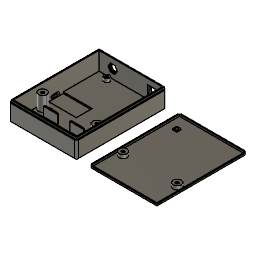
enclosure_tx (Autodesk Fusion 360 design; units mm, degrees)
part number: 2026-03-28-19-02-26-075
Autodesk Fusion 360 part; units mm, degrees
sketch "Sketch6" plane through (0, 0, 0) normal (0, 0, 1) x (1, 0, 0)
  line L0 (0, -4) -> (65, -4)
  line L1 (65, -4) -> (65, -22.2)
  line L2 (65, -22.2) -> (0, -22.2)
  line L3 (0, -22.2) -> (0, -4)
  line L4 (7.5, 70) -> (57.5, 70)
  line L5 (57.5, 70) -> (57.5, 0)
  line L6 (57.5, 0) -> (7.5, 0)
  line L7 (7.5, 0) -> (7.5, 70)
  line L8 (-5, 73) -> (70, 73)
  line L9 (70, 73) -> (70, -27)
  line L10 (70, -27) -> (-5, -27)
  line L11 (-5, -27) -> (-5, 73)
  dimension "d33" = 18.2
  dimension "d35" = 65
  dimension "d36" = 50
  dimension "d37" = 70
  dimension "d38" = 4
  dimension "d39" = 7.5
  dimension "d40" = 75
  dimension "d41" = 100
  dimension "d42" = 3
  dimension "d43" = 12.5
  constraint horizontal L0
  constraint vertical L1
  constraint horizontal L2
  constraint vertical L3
  constraint horizontal L4
  constraint vertical L5
  constraint horizontal L6
  constraint vertical L7
  constraint horizontal L8
  constraint vertical L9
  constraint horizontal L10
  constraint vertical L11
  measures "d33" distance of L0.start L2.end
  measures "d35" distance of L1.end L2.end
  measures "d36" distance of L4.start L4.end
  measures "d37" distance of L4.start L6.end
  measures "d38" distance of L0 L6
  measures "d39" distance of L3 L7
  measures "d40" distance of L8.start L8.end
  measures "d41" distance of L8.start L10.end
  measures "d42" distance of L4 L8
  measures "d43" distance of L7 L11
extrude "Extrude9" add sketch "Sketch6" along normal blind 22 contours L0 L1 L2 L3 | L4 L5 L6 L7 | L8 L9 L10 L11 makes body 1
sketch "Sketch7" plane through (0, 0, 22) normal (0, 0, 1) x (-1, 0, 0)
  line L0 (5, 27) -> (-70, 27)
  line L1 (-70, 27) -> (-70, -73)
  line L2 (-70, -73) -> (5, -73)
  line L3 (5, -73) -> (5, 27)
  line L4 (2.5, -70.5) -> (-67.5, -70.5)
  line L5 (-67.5, -70.5) -> (-67.5, 24.5)
  line L6 (-67.5, 24.5) -> (2.5, 24.5)
  line L7 (2.5, 24.5) -> (2.5, -70.5)
  line L8 (5, -73) -> (-70, -73)
  line L9 (5, 27) -> (5, -73)
  dimension "d46" = 70
  dimension "d47" = 95
  dimension "d48" = 2.5
  dimension "d49" = 2.5
  constraint horizontal L4
  constraint vertical L5
  constraint horizontal L6
  constraint vertical L7
  measures "d46" distance of L4.start L4.end
  measures "d47" distance of L4.start L6.end
  measures "d48" distance of L4 L8
  measures "d49" distance of L7 L9
extrude "Extrude10" cut sketch "Sketch7" against normal blind 20 contours L4 L5 L6 L7 bodies 1
sketch "Sketch8" plane through (0, 0, 2) normal (0, 0, 1) x (-1, 0, 0)
  line L0 (2.5, 24.5) -> (-67.5, 24.5)
  line L1 (-67.5, 24.5) -> (-67.5, -70.5)
  line L2 (-67.5, -70.5) -> (2.5, -70.5)
  line L3 (2.5, -70.5) -> (2.5, 24.5)
  line L4 (-7.5, -68.5) -> (-57.5, -68.5)
  line L5 (-57.5, -68.5) -> (-57.5, 1.5)
  line L6 (-57.5, 1.5) -> (-7.5, 1.5)
  line L7 (-7.5, 1.5) -> (-7.5, -68.5)
  line L8 (2.5, 24.5) -> (2.5, -70.5)
  line L9 (0, 4.3) -> (-65, 4.3)
  line L10 (-65, 4.3) -> (-65, 22.5)
  line L11 (-65, 22.5) -> (0, 22.5)
  line L12 (0, 22.5) -> (0, 4.3)
  line L13 (2.5, -70.5) -> (-67.5, -70.5)
  line L14 (-10.5, 3.85) -> (-25.5, 3.85)
  line L15 (-25.5, 3.85) -> (-25.5, 2.35)
  line L16 (-25.5, 2.35) -> (-10.5, 2.35)
  line L17 (-10.5, 2.35) -> (-10.5, 3.85)
  line L18 (-39.5, 2.35) -> (-54.5, 2.35)
  line L19 (-54.5, 2.35) -> (-54.5, 3.85)
  line L20 (-54.5, 3.85) -> (-39.5, 3.85)
  line L21 (-39.5, 3.85) -> (-39.5, 2.35)
  line L22 (-67.5, 24.5) -> (2.5, 24.5)
  line L23 (-25.51, 22.9) -> (-40.51, 22.9)
  line L24 (-40.51, 22.9) -> (-40.51, 24.15)
  line L25 (-40.51, 24.15) -> (-25.51, 24.15)
  line L26 (-25.51, 24.15) -> (-25.51, 22.9)
  circle A0 centre (-10.8, -65.7) radius 1.5
  circle A1 centre (-54.2, -65.7) radius 1.5
  circle A2 centre (-54.2, -1.3) radius 1.5
  circle A3 centre (-10.8, -1.3) radius 1.5
  circle A4 centre (-10.8, -65.7) radius 3
  circle A5 centre (-54.2, -65.7) radius 3
  circle A6 centre (-54.2, -1.3) radius 3
  circle A7 centre (-10.8, -1.3) radius 3
  line L27 (-65, 19.4) -> (0, 19.4)
  line L28 (0, 19.4) -> (0, 7.4)
  line L29 (0, 7.4) -> (-65, 7.4)
  line L30 (-65, 7.4) -> (-65, 19.4)
  dimension "d52" = 50
  dimension "d53" = 70
  dimension "d54" = 10
  dimension "d55" = 65
  dimension "d56" = 18.2
  dimension "d57" = 2.5
  dimension "d58" = 2
  dimension "d59" = 15
  dimension "d60" = 1.5
  dimension "d61" = 0.45
  dimension "d62" = 15
  dimension "d63" = 1.5
  dimension "d64" = 0.45
  dimension "d65" = 3
  dimension "d66" = 3
  dimension "d67" = 2
  dimension "d68" = 15
  dimension "d69" = 1.25
  dimension "d70" = 0.4
  dimension "d71" = 0.01
  dimension "d72" = 1.01
  dimension "d73" = 3
  dimension "d74" = 3
  dimension "d75" = 3
  dimension "d76" = 3
  dimension "d77" = 3.3
  dimension "d78" = 2.8
  dimension "d79" = 2.8
  dimension "d80" = 2.8
  dimension "d81" = 2.8
  dimension "d82" = 3.3
  dimension "d83" = 3.3
  dimension "d84" = 3.3
  dimension "d85" = 6
  dimension "d86" = 6
  dimension "d87" = 6
  dimension "d88" = 6
  dimension "d93" = 12
  dimension "d94" = 3.1
  constraint horizontal L4
  constraint vertical L5
  constraint horizontal L6
  constraint vertical L7
  constraint horizontal L9
  constraint vertical L10
  constraint horizontal L11
  constraint vertical L12
  constraint horizontal L14
  constraint vertical L15
  constraint horizontal L16
  constraint vertical L17
  constraint horizontal L18
  constraint vertical L19
  constraint horizontal L20
  constraint vertical L21
  constraint horizontal L23
  constraint vertical L24
  constraint horizontal L25
  constraint vertical L26
  constraint concentric A0 A4
  constraint concentric A1 A5
  constraint concentric A2 A6
  constraint concentric A3 A7
  constraint horizontal L27
  constraint vertical L28
  constraint horizontal L29
  constraint vertical L30
  constraint coincident L12 L28.end
  constraint coincident L10 L27.start
  measures "d52" distance of L4.start L4.end
  measures "d53" distance of L4.start L6.end
  measures "d54" distance of L7 L8
  measures "d55" distance of L9.start L9.end
  measures "d56" distance of L9.start L11.end
  measures "d57" distance of L8 L12
  measures "d58" distance of L4 L13
  measures "d59" distance of L14.start L14.end
  measures "d60" distance of L14.start L16.end
  measures "d61" distance of L9 L14
  measures "d62" distance of L18.start L18.end
  measures "d63" distance of L18.start L20.end
  measures "d64" distance of L9 L20
  measures "d65" distance of L5 L19
  measures "d66" distance of L7 L17
  measures "d67" distance of L11 L22
  measures "d68" distance of L23.start L23.end
  measures "d69" distance of L23.start L25.end
  measures "d70" distance of L11 L23
  measures "d71" distance of L15 L26
  measures "d72" distance of L21 L24
  measures "d73" diameter of A0
  measures "d74" diameter of A1
  measures "d75" diameter of A2
  measures "d76" diameter of A3
  measures "d77" distance of L5 A1.centre
  measures "d78" distance of L4 A1.centre
  measures "d79" distance of L4 A0.centre
  measures "d80" distance of L6 A2.centre
  measures "d81" distance of L6 A3.centre
  measures "d82" distance of L7 A0.centre
  measures "d83" distance of L7 A3.centre
  measures "d84" distance of L5 A2.centre
  measures "d85" diameter of A4
  measures "d86" diameter of A5
  measures "d87" diameter of A6
  measures "d88" diameter of A7
  measures "d93" distance of L27 L29
  measures "d94" distance of L11 L27
extrude "Extrude11" add sketch "Sketch8" along normal blind 4 contours L4 A4 | L4 A4 | L6 A7 | L6 A7 | L4 A5 | L4 A5 | L6 A6 | L6 A6 bodies 1
extrude "Extrude12" add sketch "Sketch8" along normal blind 10 contours L14 L15 L16 L17 | L18 L19 L20 L21 | L23 L24 L25 L26 bodies 1
extrude "Extrude13" cut sketch "Sketch8" against normal blind 1 contours L9 L10 L12 L29 | L10 L12 L27 L28 L29 L30 | L10 L11 L12 L27 bodies 1
fillet "Fillet1" radius 4.19 2 edges at (32.5, -4.3, 1) (32.5, -22.5, 1) on bodies 1
thread "Thread1" "ISO Metric profile 3.0 M3x0.5 M3x0.5 6H" major diameter 3.086 minor diameter 2.529 pitch 0.5 angle 60 modelled right hand crest width 0.1368 on face at (9.4178, 65.1173, 4.6667) crest through (9.5355, 65.7, 2.125) on face at (52.7464, 65.3299, 4.6667) crest through (52.9355, 65.7, 2.125) on face at (9.3075, 1.4494, 4.6667) crest through (9.5355, 1.3, 2.125) on face at (53.7223, -0.1219, 4.6667) crest through (52.9355, 1.3, 2.125) on bodies 1
sketch "Sketch9" plane through (0, 70.5, 0) normal (0, -1, 0) x (1, 0, 0)
  line L0 (67.5, 22) -> (-2.5, 22)
  line L1 (-2.5, 22) -> (-2.5, 2)
  line L2 (-2.5, 2) -> (67.5, 2)
  line L3 (67.5, 2) -> (67.5, 22)
  line L4 (10, 7.5) -> (15, 7.5)
  line L5 (15, 7.5) -> (17.5, 11.8301)
  line L6 (17.5, 11.8301) -> (15, 16.1603)
  line L7 (15, 16.1603) -> (10, 16.1603)
  line L8 (10, 16.1603) -> (7.5, 11.8301)
  line L9 (7.5, 11.8301) -> (10, 7.5)
  line L10 (10, 7.5) -> (15, 7.5) construction
  circle A0 centre (12.5, 11.8301) radius 3.25
  line L11 (51.1, 15.9) -> (59.5, 15.9)
  line L12 (59.5, 15.9) -> (59.5, 7.5)
  line L13 (59.5, 7.5) -> (51.1, 7.5)
  line L14 (51.1, 7.5) -> (51.1, 15.9)
  line L15 (53.1, 13.9) -> (57.5, 13.9)
  line L16 (57.5, 13.9) -> (57.5, 9.5)
  line L17 (57.5, 9.5) -> (53.1, 9.5)
  line L18 (53.1, 9.5) -> (53.1, 13.9)
  point P0 (12.5, 11.8301)
  dimension "d101" = 5
  dimension "d102" = 0
  dimension "d103" = 6.5
  dimension "d104" = 15
  dimension "d105" = 8.4
  dimension "d106" = 8.4
  dimension "d107" = 4.4
  dimension "d108" = 4.4
  dimension "d109" = 2
  dimension "d110" = 2
  dimension "d111" = 5.5
  dimension "d112" = 5.5
  dimension "d113" = 8
  constraint horizontal L10
  constraint coincident P0 A0.centre
  constraint horizontal L11
  constraint vertical L12
  constraint horizontal L13
  constraint vertical L14
  constraint horizontal L15
  constraint vertical L16
  constraint horizontal L17
  constraint vertical L18
  measures "d101" distance of L4.start L4.end
  measures "d102" angle of L4 L10
  measures "d103" diameter of A0
  measures "d104" distance of L1 P0
  measures "d105" distance of L11.start L11.end
  measures "d106" distance of L11.start L13.end
  measures "d107" distance of L15.start L15.end
  measures "d108" distance of L15.start L17.end
  measures "d109" distance of L11 L15
  measures "d110" distance of L12 L16
  measures "d111" distance of L2 L4
  measures "d112" distance of L2 L13
  measures "d113" distance of L3 L12
extrude "Extrude14" cut sketch "Sketch9" against normal blind 1.2 contours L4 L5 L6 L7 L8 L9 bodies 1
extrude "Extrude15" cut sketch "Sketch9" against normal blind 10 contours A0 bodies 1
extrude "Extrude16" cut sketch "Sketch9" against normal blind 1.8 contours L11 L12 L13 L14 bodies 1
extrude "Extrude17" cut sketch "Sketch9" against normal blind 10 contours L15 L16 L17 L18 bodies 1
sketch "Sketch10" plane through (0, 0, 2) normal (0, 0, 1) x (-1, 0, 0)
  line L0 (0, 4.3) -> (-65, 4.3)
  line L1 (-65, 4.3) -> (-65, 22.5)
  line L2 (-65, 22.5) -> (0, 22.5)
  line L3 (0, 22.5) -> (0, 4.3)
  line L4 (-25.51, 24.15) -> (-25.51, 22.9)
  line L5 (-25.51, 22.9) -> (-40.51, 22.9)
  line L6 (-40.51, 22.9) -> (-40.51, 24.15)
  line L7 (-40.51, 24.15) -> (-25.51, 24.15)
  line L8 (-39.5, 3.85) -> (-39.5, 2.35)
  line L9 (-39.5, 2.35) -> (-54.5, 2.35)
  line L10 (-54.5, 2.35) -> (-54.5, 3.85)
  line L11 (-54.5, 3.85) -> (-39.5, 3.85)
  line L12 (-10.5, 2.35) -> (-25.5, 2.35)
  line L13 (-25.5, 2.35) -> (-25.5, 3.85)
  line L14 (-25.5, 3.85) -> (-10.5, 3.85)
  line L15 (-10.5, 3.85) -> (-10.5, 2.35)
  circle A0 centre (-10.8, -65.7) radius 3
  circle A1 centre (-54.2, -65.7) radius 3
  line L16 (2.5, 24.5) -> (-67.5, 24.5)
  line L17 (-67.5, 24.5) -> (-67.5, -70.5)
  line L18 (-67.5, -70.5) -> (2.5, -70.5)
  line L19 (2.5, -70.5) -> (2.5, 24.5)
  circle A2 centre (-54.2, -1.3) radius 3
  circle A3 centre (-10.8, -1.3) radius 3
  line L20 (2.5, -13.3) -> (-29.5, -13.3)
  line L21 (-29.5, -13.3) -> (-29.5, -30.8)
  line L22 (-29.5, -30.8) -> (2.5, -30.8)
  line L23 (2.5, -30.8) -> (2.5, -13.3)
  dimension "d122" = 32
  dimension "d123" = 17.5
  dimension "d126" = 12
  constraint horizontal L20
  constraint vertical L21
  constraint horizontal L22
  constraint vertical L23
  constraint coincident L19 L20.start
  measures "d122" distance of L20.start L20.end
  measures "d123" distance of L20.start L22.end
  measures "d126" distance of A3.centre L20
extrude "Extrude18" cut sketch "Sketch10" against normal blind 1.5 contours L19 L20 L21 L22 L23 bodies 1
sketch "Sketch11" plane through (-2.5, 0, 0) normal (1, 0, 0) x (0, 1, 0)
  line L0 (70.5, 22) -> (-24.5, 22)
  line L1 (-24.5, 22) -> (-24.5, 2)
  line L2 (-24.5, 2) -> (13.3, 2)
  line L3 (13.3, 2) -> (13.3, 0.5)
  line L4 (13.3, 0.5) -> (30.8, 0.5)
  line L5 (30.8, 0.5) -> (30.8, 2)
  line L6 (30.8, 2) -> (70.5, 2)
  line L7 (70.5, 2) -> (70.5, 22)
  line L8 (30.8, 0.5) -> (13.3, 0.5)
  line L9 (13.3, 0.5) -> (13.3, 6.5)
  line L10 (13.3, 6.5) -> (30.8, 6.5)
  line L11 (30.8, 6.5) -> (30.8, 0.5)
  line L12 (18.95, 1.7) -> (25.15, 1.7)
  arc A0 (25.15, 1.7) -> (25.15, 4.9) centre (25.15, 3.3) ccw
  line L13 (25.15, 4.9) -> (18.95, 4.9)
  arc A1 (18.95, 4.9) -> (18.95, 1.7) centre (18.95, 3.3) ccw
  line L14 (18.95, 3.3) -> (25.15, 3.3) construction
  dimension "d127" = 17.5
  dimension "d128" = 6
  dimension "d129" = 6.2
  dimension "d130" = 1.6
  dimension "d131" = 1.2
  dimension "d132" = 5.65
  constraint horizontal L8
  constraint vertical L9
  constraint horizontal L10
  constraint vertical L11
  constraint coincident L4.end L5.start
  constraint tangent L12 A0
  constraint tangent A0 L13
  constraint parallel L12 L13
  constraint tangent L13 A1
  constraint tangent L12 A1
  constraint horizontal L14
  measures "d127" distance of L4.end L3.end
  measures "d128" distance of L4.end L10.end
  measures "d129" distance of A1.centre A0.centre
  measures "d130" radius of A0
  measures "d131" distance of L8 L12
  measures "d132" distance of L9 A1.centre
extrude "Extrude19" cut sketch "Sketch11" against normal blind 5 contours L12 A0 L13 A1 bodies 1
sketch "Sketch12" plane through (0, 0, 22) normal (0, 0, 1) x (-1, 0, 0)
  line L0 (-67.5, -70.5) -> (-67.5, 24.5)
  line L1 (-67.5, 24.5) -> (2.5, 24.5)
  line L2 (2.5, 24.5) -> (2.5, -70.5)
  line L3 (2.5, -70.5) -> (-67.5, -70.5)
  line L4 (5, 27) -> (-70, 27)
  line L5 (-70, 27) -> (-70, -73)
  line L6 (-70, -73) -> (5, -73)
  line L7 (5, -73) -> (5, 27)
  line L8 (-68.75, 25.75) -> (3.75, 25.75)
  line L9 (3.75, 25.75) -> (3.75, -71.75)
  line L10 (3.75, -71.75) -> (-68.75, -71.75)
  line L11 (-68.75, -71.75) -> (-68.75, 25.75)
  dimension "d135" = 72.5
  dimension "d136" = 97.5
  dimension "d137" = 1.25
  dimension "d138" = 1.25
  constraint horizontal L8
  constraint vertical L9
  constraint horizontal L10
  constraint vertical L11
  measures "d135" distance of L8.start L8.end
  measures "d136" distance of L8.start L10.end
  measures "d137" distance of L1 L8
  measures "d138" distance of L0 L11
extrude "Extrude20" cut sketch "Sketch12" against normal blind 2 contours L4 L5 L6 L7 bodies 1
sketch "Sketch13" plane through (0, 0, 0) normal (0, 0, 1) x (1, 0, 0)
  line L0 (83.9922, 73.0345) -> (158.9922, 73.0345)
  line L1 (158.9922, 73.0345) -> (158.9922, -26.9655)
  line L2 (158.9922, -26.9655) -> (83.9922, -26.9655)
  line L3 (83.9922, -26.9655) -> (83.9922, 73.0345)
  dimension "d141" = 75
  dimension "d142" = 100
  constraint horizontal L0
  constraint vertical L1
  constraint horizontal L2
  constraint vertical L3
  measures "d141" distance of L0.start L0.end
  measures "d142" distance of L0.start L2.end
extrude "Extrude21" add sketch "Sketch13" along normal blind 4 separate body makes body 2
sketch "Sketch14" plane through (0, 0, 4) normal (0, 0, 1) x (-1, 0, 0)
  line L0 (-83.9922, 26.9655) -> (-158.9922, 26.9655)
  line L1 (-158.9922, 26.9655) -> (-158.9922, -73.0345)
  line L2 (-158.9922, -73.0345) -> (-83.9922, -73.0345)
  line L3 (-83.9922, -73.0345) -> (-83.9922, 26.9655)
  line L4 (-85.2422, -71.7845) -> (-157.7422, -71.7845)
  line L5 (-157.7422, -71.7845) -> (-157.7422, 25.7155)
  line L6 (-157.7422, 25.7155) -> (-85.2422, 25.7155)
  line L7 (-85.2422, 25.7155) -> (-85.2422, -71.7845)
  dimension "d145" = 72.5
  dimension "d146" = 97.5
  dimension "d147" = 1.25
  dimension "d148" = 1.25
  constraint horizontal L4
  constraint vertical L5
  constraint horizontal L6
  constraint vertical L7
  measures "d145" distance of L4.start L4.end
  measures "d146" distance of L4.start L6.end
  measures "d147" distance of L2 L4
  measures "d148" distance of L3 L7
sketch "Sketch15" plane through (0, 0, 4) normal (0, 0, 1) x (-1, 0, 0)
  line L0 (-86.4922, -70.5345) -> (-156.4922, -70.5345)
  line L1 (-156.4922, -70.5345) -> (-156.4922, 24.4655)
  line L2 (-156.4922, 24.4655) -> (-86.4922, 24.4655)
  line L3 (-86.4922, 24.4655) -> (-86.4922, -70.5345)
  line L4 (-85.2422, -71.7845) -> (-157.7422, -71.7845)
  line L5 (-85.2422, 25.7155) -> (-85.2422, -71.7845)
  dimension "d149" = 70
  dimension "d150" = 95
  dimension "d151" = 1.25
  dimension "d152" = 1.25
  constraint horizontal L0
  constraint vertical L1
  constraint horizontal L2
  constraint vertical L3
  measures "d149" distance of L0.start L0.end
  measures "d150" distance of L0.start L2.end
  measures "d151" distance of L0 L4
  measures "d152" distance of L3 L5
extrude "Extrude23" cut sketch "Sketch14" against normal blind 2 contours L4 L5 L6 L7 bodies 2
sketch "Sketch16" plane through (0, 0, 2) normal (0, 0, 1) x (-1, 0, 0)
  circle A0 centre (-10.8, -1.3) radius 3
  circle A1 centre (-54.2, -1.3) radius 3
  line L0 (2.5, -30.8) -> (-29.5, -30.8)
  line L1 (-29.5, -30.8) -> (-29.5, -13.3)
  line L2 (-29.5, -13.3) -> (2.5, -13.3)
  line L3 (2.5, -13.3) -> (2.5, 24.5)
  line L4 (2.5, 24.5) -> (-67.5, 24.5)
  line L5 (-67.5, 24.5) -> (-67.5, -70.5)
  line L6 (-67.5, -70.5) -> (2.5, -70.5)
  line L7 (2.5, -70.5) -> (2.5, -30.8)
  circle A2 centre (-54.2, -65.7) radius 3
  circle A3 centre (-10.8, -65.7) radius 3
  line L8 (-10.5, 2.35) -> (-25.5, 2.35)
  line L9 (-25.5, 2.35) -> (-25.5, 3.85)
  line L10 (-25.5, 3.85) -> (-10.5, 3.85)
  line L11 (-10.5, 3.85) -> (-10.5, 2.35)
  line L12 (-39.5, 3.85) -> (-39.5, 2.35)
  line L13 (-39.5, 2.35) -> (-54.5, 2.35)
  line L14 (-54.5, 2.35) -> (-54.5, 3.85)
  line L15 (-54.5, 3.85) -> (-39.5, 3.85)
  line L16 (-25.51, 24.15) -> (-25.51, 22.9)
  line L17 (-25.51, 22.9) -> (-40.51, 22.9)
  line L18 (-40.51, 22.9) -> (-40.51, 24.15)
  line L19 (-40.51, 24.15) -> (-25.51, 24.15)
  line L20 (0, 4.3) -> (-65, 4.3)
  line L21 (-65, 4.3) -> (-65, 22.5)
  line L22 (-65, 22.5) -> (0, 22.5)
  line L23 (0, 22.5) -> (0, 4.3)
  line L24 (0, -5.5) -> (-5, -5.5)
  line L25 (-5, -5.5) -> (-5, -0.5)
  line L26 (-5, -0.5) -> (0, -0.5)
  line L27 (0, -0.5) -> (0, -5.5)
  line L28 (-60, -5.5) -> (-65, -5.5)
  line L29 (-65, -5.5) -> (-65, -0.5)
  line L30 (-65, -0.5) -> (-60, -0.5)
  line L31 (-60, -0.5) -> (-60, -5.5)
  line L32 (3.75, -71.75) -> (3.75, 25.75)
  line L33 (-68.75, 25.75) -> (-68.75, -71.75)
  line L34 (-85.2422, 25.7155) -> (-85.2422, -71.7845)
  line L35 (-157.7422, -71.7845) -> (-157.7422, 25.7155)
  circle A4 centre (-2.5, -3) radius 1.5
  circle A5 centre (-62.5, -3) radius 1.5
  circle A6 centre (-91.4922, -3.0345) radius 1.25
  circle A7 centre (-151.4922, -3.0345) radius 1.5
  circle A8 centre (-2.5, -3) radius 4.5
  circle A9 centre (-62.5, -3) radius 4.5
  circle A10 centre (-151.4922, -3.0345) radius 4.5
  circle A11 centre (-91.4922, -3.0345) radius 4.5
  line L36 (-83.9922, 26.9655) -> (-158.9922, 26.9655)
  line L37 (-70, 27) -> (5, 27)
  dimension "d157" = 3.75
  dimension "d158" = 3.75
  dimension "d161" = 3
  dimension "d162" = 2.5
  dimension "d163" = 2.5
  dimension "d164" = 3
  dimension "d165" = 2.5
  dimension "d166" = 2.5
  dimension "d167" = 2.5
  dimension "d170" = 3
  dimension "d183" = 9
  dimension "d184" = 9
  dimension "d211" = 9
  dimension "d212" = 9
  dimension "d213" = 30
  dimension "d214" = 30
  dimension "d215" = 30
  dimension "d216" = 30
  constraint horizontal L24
  constraint vertical L25
  constraint horizontal L26
  constraint vertical L27
  constraint horizontal L28
  constraint vertical L29
  constraint horizontal L30
  constraint vertical L31
  constraint concentric A4 A8
  constraint concentric A5 A9
  constraint concentric A7 A10
  constraint concentric A6 A11
  measures "d157" distance of L27 L32
  measures "d158" distance of L29 L33
  measures "d161" diameter of A4
  measures "d162" distance of L24 A4.centre
  measures "d163" distance of L25 A4.centre
  measures "d164" diameter of A5
  measures "d165" distance of L30 A5.centre
  measures "d166" distance of L29 A5.centre
  measures "d167" diameter of A6
  measures "d170" diameter of A7
  measures "d183" diameter of A8
  measures "d184" diameter of A9
  measures "d211" diameter of A10
  measures "d212" diameter of A11
  measures "d213" distance of A7.centre L36
  measures "d214" distance of A6.centre L36
  measures "d215" distance of A5.centre L37
  measures "d216" distance of A4.centre L37
extrude "Extrude25" add sketch "Sketch16" along normal blind 4 contours A10 | A11 bodies 2
sketch "Sketch17" plane through (0, 0, 0) normal (0, 0, -1) x (1, 0, 0)
  line L0 (70, 27) -> (-5, 27)
  line L1 (-5, 27) -> (-5, -73)
  line L2 (-5, -73) -> (70, -73)
  line L3 (70, -73) -> (70, 27)
  circle A0 centre (62.5375, -2.8213) radius 3.1
  circle A1 centre (2.5, -3) radius 3.1
  dimension "d219" = 6.2
  dimension "d220" = 6.2
  measures "d219" diameter of A0
  measures "d220" diameter of A1
extrude "Extrude29" add sketch "Sketch16" along normal blind 16 contours L24 L25 L26 L27 | L28 L29 L30 L31 | A4 | A5 | A8 | A9 bodies 1
sketch "Sketch18" plane through (0, 0, 18) normal (0, 0, 1) x (-1, 0, 0)
  circle A0 centre (-2.5, -3) radius 4.5
  circle A1 centre (-62.5, -3) radius 1.5
  line L0 (-65, -0.5) -> (-60, -0.5)
  line L1 (-60, -0.5) -> (-60, -5.5)
  line L2 (-60, -5.5) -> (-65, -5.5)
  line L3 (-65, -5.5) -> (-65, -0.5)
  circle A2 centre (-2.5, -3) radius 1.5
  line L4 (-5, -0.5) -> (0, -0.5)
  line L5 (0, -0.5) -> (0, -5.5)
  line L6 (0, -5.5) -> (-5, -5.5)
  line L7 (-5, -5.5) -> (-5, -0.5)
  dimension "d217" = 3
  dimension "d218" = 3
  constraint horizontal L0
  constraint vertical L1
  constraint horizontal L2
  constraint vertical L3
  constraint concentric A0 A2
  constraint horizontal L4
  constraint vertical L5
  constraint horizontal L6
  constraint vertical L7
  measures "d217" diameter of A1
  measures "d218" diameter of A2
extrude "Extrude32" cut sketch "Sketch18" against normal blind 25 contours A1 | A2 bodies 1
extrude "Extrude33" cut sketch "Sketch17" against normal blind 12 contours A0 | A1 bodies 1
sketch "Sketch19" plane through (0, 0, 2) normal (0, 0, 1) x (-1, 0, 0)
  line L0 (-85.2422, 25.7155) -> (-157.7422, 25.7155)
  line L1 (-157.7422, 25.7155) -> (-157.7422, -71.7845)
  line L2 (-157.7422, -71.7845) -> (-85.2422, -71.7845)
  line L3 (-85.2422, -71.7845) -> (-85.2422, 25.7155)
  line L4 (-93.9922, -60) -> (-98.9922, -60)
  line L5 (-98.9922, -60) -> (-98.9922, -55)
  line L6 (-98.9922, -55) -> (-93.9922, -55)
  line L7 (-93.9922, -55) -> (-93.9922, -60)
  circle A0 centre (-96.4922, -57.5) radius 1.5
  line L8 (-83.9922, -73.0345) -> (-83.9922, 26.9655)
  circle A1 centre (-91.4922, -3.0345) radius 4.5
  circle A2 centre (-151.4922, -3.0345) radius 4.5
  dimension "d201" = 5
  dimension "d202" = 5
  dimension "d203" = 3
  dimension "d204" = 2.5
  dimension "d205" = 2.5
  dimension "d206" = 10
  constraint horizontal L4
  constraint vertical L5
  constraint horizontal L6
  constraint vertical L7
  measures "d201" distance of L4.start L4.end
  measures "d202" distance of L4.start L6.end
  measures "d203" diameter of A0
  measures "d204" distance of L4 A0.centre
  measures "d205" distance of L7 A0.centre
  measures "d206" distance of L7 L8
extrude "Extrude34" cut sketch "Sketch19" against normal blind 2.5 contours A0 bodies 2
extrude "Extrude35" add sketch "Sketch19" along normal blind 0.6 contours L4 L5 L6 L7 bodies 2
thread "Thread3" "ISO Metric profile 3.0 M3x0.5 M3x0.5 6H" major diameter 3.086 minor diameter 2.529 pitch 0.5 angle 60 modelled right hand crest width 0.1368 on face at (1.0075, 3.1494, 16) crest through (1.2355, 3, 17.875) on face at (63.1843, 4.3348, 16) crest through (61.2355, 3, 17.875) on face at (152.1091, 1.6672, 4.6667) crest through (150.2277, 3.0345, 2.125) on face at (91.0941, 1.8496, 4.6667) crest through (90.2277, 3.0345, 2.125) on bodies 1 2
chamfer "Chamfer1" distance 2.2 angle 45 16 edges at (-5, -27, 10) (70, -27, 10) (70, 73, 10) (-5, 73, 10) (-5, 23, 0) (32.5, -27, 0) (70, 23, 0) (32.5, 73, 0) (83.9922, 23.0345, 0) (121.4922, -26.9655, 0) (83.9922, -26.9655, 2) (83.9922, 73.0345, 2) (121.4922, 73.0345, 0) (158.9922, 73.0345, 2) (158.9922, 23.0345, 0) (158.9922, -26.9655, 2) on bodies 1 2
